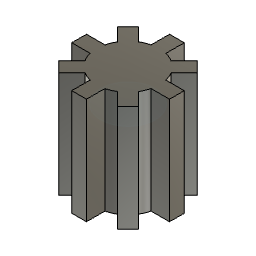
sprocket v7 (Autodesk Fusion 360 design; units mm, degrees)
Autodesk Fusion 360 part; units mm, degrees
note: some values were not read from the file. Set by a fixed rule: which sketch regions a step uses.
sketch "Sketch1" plane through (0, 0, 0) normal (0, 0, 1) x (1, 0, 0)
  circle A0 centre (0, 0) radius 4.25
  line L0 (1.0019, 4.1311) -> (1.0019, 6.6311)
  line L1 (1.0019, 6.6311) -> (-0.9981, 6.6311)
  line L2 (-0.9981, 6.6311) -> (-0.9981, 4.1311)
  line L3 (-5.3947, 3.9831) -> (-3.6269, 2.2154)
  line L4 (-3.9805, 5.3974) -> (-5.3947, 3.9831)
  line L5 (-2.2127, 3.6296) -> (-3.9805, 5.3974)
  line L6 (-6.6311, -0.9981) -> (-4.1311, -0.9981)
  line L7 (-6.6311, 1.0019) -> (-6.6311, -0.9981)
  line L8 (-4.1311, 1.0019) -> (-6.6311, 1.0019)
  line L9 (-3.9831, -5.3947) -> (-2.2154, -3.6269)
  line L10 (-5.3974, -3.9805) -> (-3.9831, -5.3947)
  line L11 (-3.6296, -2.2127) -> (-5.3974, -3.9805)
  line L12 (0.9981, -6.6311) -> (0.9981, -4.1311)
  line L13 (-1.0019, -6.6311) -> (0.9981, -6.6311)
  line L14 (-1.0019, -4.1311) -> (-1.0019, -6.6311)
  line L15 (5.3947, -3.9831) -> (3.6269, -2.2154)
  line L16 (3.9805, -5.3974) -> (5.3947, -3.9831)
  line L17 (2.2127, -3.6296) -> (3.9805, -5.3974)
  line L18 (6.6311, 0.9981) -> (4.1311, 0.9981)
  line L19 (6.6311, -1.0019) -> (6.6311, 0.9981)
  line L20 (4.1311, -1.0019) -> (6.6311, -1.0019)
  line L21 (3.9831, 5.3947) -> (2.2154, 3.6269)
  line L22 (5.3974, 3.9805) -> (3.9831, 5.3947)
  line L23 (3.6296, 2.2127) -> (5.3974, 3.9805)
  line L24 (-2.2127, 3.6296) -> (-0.9981, 4.1311)
  line L25 (1.0019, 4.1311) -> (2.2154, 3.6269)
  line L26 (3.6296, 2.2127) -> (4.1311, 0.9981)
  line L27 (4.1311, -1.0019) -> (3.6269, -2.2154)
  line L28 (2.2127, -3.6296) -> (0.9981, -4.1311)
  line L29 (-1.0019, -4.1311) -> (-2.2154, -3.6269)
  line L30 (-3.6296, -2.2127) -> (-4.1311, -0.9981)
  line L31 (-4.1311, 1.0019) -> (-3.6269, 2.2154)
  line L32 (-2.2127, 3.6296) -> (-0.9981, 4.1311)
  point P0 (-0.9981, 4.1311)
  dimension "d1" = 8.5
  dimension "d3" = 2
  dimension "d5" = 360
  constraint coincident A0.centre origin
  constraint vertical L0
  constraint horizontal L1
  constraint vertical L2
  constraint coincident A0 P0
  constraint coincident P0 L2.end
  constraint parallel L24 L32
  measures "d1" diameter of A0
  measures "d3" distance of L0 L2
extrude "Extrude1" add sketch "Sketch1" along normal blind 14.4 contours A0 L24 L25 L26 L27 L28 L29 L30 L31 L32 | A0 L26 | A0 L27 | A0 L25 | A0 L28 | A0 L24 L32 | A0 L29 | A0 L31 | A0 L30 makes body 1
delete_body "RemoveBody1" bodies 1
sketch "Sketch2" plane through (0, 0, 0) normal (0, 0, 1) x (1, 0, 0)
  line L0 (-0.9981, 4.1311) -> (1.0019, 4.1311)
  line L1 (2.2154, 3.6269) -> (3.6296, 2.2127)
  line L2 (4.1311, 0.9981) -> (4.1311, -1.0019)
  line L3 (2.2127, -3.6296) -> (3.6269, -2.2154)
  line L4 (-1.0019, -4.1311) -> (0.9981, -4.1311)
  line L5 (-3.6296, -2.2127) -> (-2.2154, -3.6269)
  line L6 (-4.1311, 1.0019) -> (-4.1311, -0.9981)
  line L7 (-2.2127, 3.6296) -> (-3.6182, 2.2448)
  point P0 (-0.9981, 4.1311)
  point P1 (1.0019, 4.1311)
  point P2 (2.2154, 3.6269)
  point P3 (3.6296, 2.2127)
  point P4 (4.1311, 0.9981)
  point P5 (4.1311, -1.0019)
  point P6 (2.2127, -3.6296)
  point P7 (3.6269, -2.2154)
  point P8 (-1.0019, -4.1311)
  point P9 (0.9981, -4.1311)
  point P10 (-3.6296, -2.2127)
  point P11 (-2.2154, -3.6269)
  point P12 (-4.1311, 1.0019)
  point P13 (-4.1311, -0.9981)
  point P14 (-2.2127, 3.6296)
  constraint coincident P0 L0.start
  constraint coincident P1 L0.end
  constraint coincident P2 L1.start
  constraint coincident P3 L1.end
  constraint coincident P4 L2.start
  constraint coincident P5 L2.end
  constraint coincident P6 L3.start
  constraint coincident P7 L3.end
  constraint coincident P8 L4.start
  constraint coincident P9 L4.end
  constraint coincident P10 L5.start
  constraint coincident P11 L5.end
  constraint coincident P12 L6.start
  constraint coincident P13 L6.end
  constraint coincident P14 L7.start
extrude "Extrude2" add sketch "Sketch1" along normal blind 14.4 separate body makes body 2
cylinder "CylinderPrimitive1" add diameter 7.4 height 10 placed x (1, 0, 0) y (0, 1, 0) z (0, 0, 1) at (0, 0, 0) separate body makes body 3
sketch "Sketch5" plane through (0, 0, 10) normal (0, 0, 1) x (-1, 0, 0)
  circle A0 centre (0, 0) radius 3.7
hidden bodies 3
named bodies: "sprocket"
